Housing v6 (Autodesk Fusion 360 design; units mm, degrees)
Autodesk Fusion 360 part; units mm, degrees
sketch "Sketch1" plane through (0, 0, 0) normal (0, 0, 1) x (1, 0, 0)
  circle A0 centre (0, 0) radius 42 construction
  line L0 (0, 0) -> (0, 42) construction
  circle A1 centre (0, 42) radius 2.25
  circle A2 centre (-17.0829, 38.3689) radius 2.25
  circle A3 centre (-31.2121, 28.1035) radius 2.25
  circle A4 centre (-39.9444, 12.9787) radius 2.25
  circle A5 centre (-41.7699, -4.3902) radius 2.25
  circle A6 centre (-36.3731, -21) radius 2.25
  circle A7 centre (-24.687, -33.9787) radius 2.25
  circle A8 centre (-8.7323, -41.0822) radius 2.25
  circle A9 centre (8.7323, -41.0822) radius 2.25
  circle A10 centre (24.687, -33.9787) radius 2.25
  circle A11 centre (36.3731, -21) radius 2.25
  circle A12 centre (41.7699, -4.3902) radius 2.25
  circle A13 centre (39.9444, 12.9787) radius 2.25
  circle A14 centre (31.2121, 28.1035) radius 2.25
  circle A15 centre (17.0829, 38.3689) radius 2.25
  circle A16 centre (0, 42) radius 3 construction
  circle A17 centre (-17.0829, 38.3689) radius 3 construction
  circle A18 centre (-31.2121, 28.1035) radius 3 construction
  circle A19 centre (-39.9444, 12.9787) radius 3 construction
  circle A20 centre (-41.7699, -4.3902) radius 3 construction
  circle A21 centre (-36.3731, -21) radius 3 construction
  circle A22 centre (-24.687, -33.9787) radius 3 construction
  circle A23 centre (-8.7323, -41.0822) radius 3 construction
  circle A24 centre (8.7323, -41.0822) radius 3 construction
  circle A25 centre (24.687, -33.9787) radius 3 construction
  circle A26 centre (36.3731, -21) radius 3 construction
  circle A27 centre (41.7699, -4.3902) radius 3 construction
  circle A28 centre (39.9444, 12.9787) radius 3 construction
  circle A29 centre (31.2121, 28.1035) radius 3 construction
  circle A30 centre (17.0829, 38.3689) radius 3 construction
  circle A31 centre (0, 0) radius 46
  circle A32 centre (0, 0) radius 49
  dimension "d1" = 84
  dimension "d2" = 4.5
  dimension "d4" = 360
  dimension "d5" = 6
  dimension "d7" = 360
  dimension "d8" = 92
  dimension "d9" = 3
  constraint coincident A0.centre L0.start
  constraint coincident A0 L0.end
  constraint vertical L0
  constraint coincident L0.end A1.centre
  constraint concentric A1 A16
  constraint concentric A0 A31
  measures "d1" diameter of A0
  measures "d2" diameter of A1
  measures "d5" diameter of A16
  measures "d8" diameter of A31
extrude "Extrude1" add sketch "Sketch1" along normal blind 26 contours A32
sketch "Sketch2" plane through (0, 0, 26) normal (0, 0, 1) x (-1, 0, 0)
  circle A0 centre (0, 0) radius 46
  circle A1 centre (0, 0) radius 49
  line L0 (0, 0) -> (-69, 0) construction
  line L1 (0, 0) -> (0, -46) construction
  line L2 (-48.7442, -5) -> (-60, -5)
  line L3 (-60, -5) -> (-60, 5)
  line L4 (-60, 5) -> (-48.7442, 5)
  circle A2 centre (-54, 0) radius 2.75
  line L5 (48.7442, -5) -> (60, -5)
  line L6 (60, -5) -> (60, 5)
  line L7 (60, 5) -> (48.7442, 5)
  circle A3 centre (54, 0) radius 2.75
  dimension "d12" = 5.5
  dimension "d13" = 54
  dimension "d14" = 6
  dimension "d15" = 10
  constraint coincident A0.centre A1.centre
  constraint horizontal L0
  constraint coincident A0 L1.end
  constraint perpendicular L0 L1
  constraint coincident A1 L2.start
  constraint parallel L0 L2
  constraint perpendicular L0 L3
  constraint coincident A1 L4.end
  constraint perpendicular L3 L4
  constraint coincident L0 A2.centre
  constraint symmetric L0 L2 L4
  constraint symmetric L1 L2.start L5.start
  constraint symmetric L1 L2.end L5.end
  constraint symmetric L1 L3.end L6.end
  constraint symmetric L1 L4.end L7.end
  constraint symmetric L1 A2 A3
  measures "d12" diameter of A2
  measures "d13" distance of A0.centre A2.centre
  measures "d14" distance of L3 A2.centre
  measures "d15" distance of L2.end L3.end
extrude "Extrude2" add sketch "Sketch2" against normal blind 26 contours A1 L5 L6 L7 | A1 L2 L3 L4
